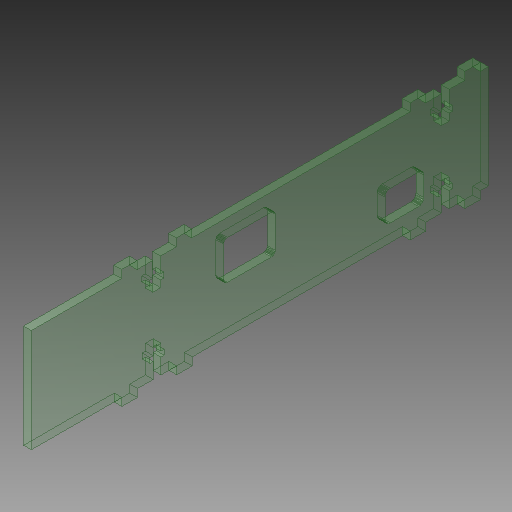
# Autodesk Inventor part: EE Side
Saved by Autodesk Inventor 2018 (Build 220112000, 112)
## iProperties
Created: 2016-07-27
Part Number: EE Side
Material: Polycarbonate, Green
Document SubType Name: Modeling
Designer: User
Density: 1.2 g/cm^3
Appearance: Polycarbonate - Clear(2)
Author: User
Autodesk Inventor part; units mm, degrees
ref_plane "YZ Plane" through (0, 0, 0) normal (1, 0, 0) x (0, 1, 0)
ref_plane "XZ Plane" through (0, 0, 0) normal (0, 1, 0) x (-1, 0, 0)
ref_plane "XY Plane" through (0, 0, 0) normal (0, 0, 1) x (1, 0, 0)
sketch "Sketch1" plane through (0, 0, 0) normal (1, 0, 0) x (0, 1, 0)
  line L0 (104.8297, -51.6375) -> (104.8297, -45.5375)
  line L1 (104.8297, -45.5375) -> (107.8297, -45.5375)
  line L2 (107.8297, -45.5375) -> (107.8297, -39.5375)
  line L3 (107.8297, -39.5375) -> (104.8297, -39.5375)
  line L4 (104.8297, -39.5375) -> (104.8297, -4.6192)
  line L5 (104.8297, -4.6192) -> (64.8298, -4.6192)
  line L6 (64.8298, -4.6192) -> (64.8298, -39.7122)
  line L7 (64.8298, -39.7122) -> (61.8297, -39.7122)
  line L8 (61.8297, -39.7122) -> (61.8297, -45.7122)
  line L9 (61.8297, -45.7122) -> (64.8298, -45.7122)
  line L10 (64.8298, -45.7122) -> (64.8298, -51.8122)
  line L11 (64.8298, -51.8122) -> (70.8298, -51.8122)
  line L12 (70.8298, -51.8122) -> (70.8298, -50.5622)
  line L13 (70.8298, -50.5622) -> (72.8298, -50.5622)
  line L14 (72.8298, -50.5622) -> (72.8298, -51.8122)
  line L15 (72.8298, -51.8122) -> (75.4798, -51.8122)
  line L16 (75.4798, -51.8122) -> (75.4798, -54.8122)
  line L17 (75.4798, -54.8122) -> (72.8298, -54.8122)
  line L18 (72.8298, -54.8122) -> (72.8298, -56.0622)
  line L19 (72.8298, -56.0622) -> (70.8298, -56.0622)
  line L20 (70.8298, -56.0622) -> (70.8298, -54.8122)
  line L21 (70.8298, -54.8122) -> (64.8298, -54.8122)
  line L22 (64.8298, -54.8122) -> (64.8298, -60.9122)
  line L23 (64.8298, -60.9122) -> (61.8297, -60.9122)
  line L24 (61.8297, -60.9122) -> (61.8297, -66.9122)
  line L25 (61.8297, -66.9122) -> (64.8298, -66.9192)
  line L26 (64.8298, -66.9192) -> (64.8298, -67.0192)
  line L27 (64.8298, -67.0192) -> (64.8298, -151.3192)
  line L28 (64.8298, -151.3192) -> (61.8297, -151.3192)
  line L29 (61.8297, -151.3192) -> (61.8297, -157.3192)
  line L30 (61.8297, -157.3192) -> (64.8298, -157.3192)
  line L31 (64.8298, -157.3192) -> (64.8298, -163.4192)
  line L32 (64.8298, -163.4192) -> (70.8298, -163.4192)
  line L33 (70.8298, -163.4192) -> (70.8298, -162.1692)
  line L34 (70.8298, -162.1692) -> (72.8298, -162.1692)
  line L35 (72.8298, -162.1692) -> (72.8298, -163.4192)
  line L36 (72.8298, -163.4192) -> (75.4798, -163.4192)
  line L37 (75.4798, -163.4192) -> (75.4798, -166.4192)
  line L38 (75.4798, -166.4192) -> (72.8298, -166.4192)
  line L39 (72.8298, -166.4192) -> (72.8298, -167.6692)
  line L40 (72.8298, -167.6692) -> (70.8298, -167.6692)
  line L41 (70.8298, -167.6692) -> (70.8298, -166.4192)
  line L42 (70.8298, -166.4192) -> (64.8298, -166.4192)
  line L43 (64.8298, -166.4192) -> (64.8298, -172.5192)
  line L44 (64.8298, -172.5192) -> (61.8297, -172.5192)
  line L45 (61.8297, -172.5192) -> (61.8297, -178.5192)
  line L46 (61.8297, -178.5192) -> (64.8298, -178.5192)
  line L47 (64.8298, -178.5192) -> (64.8298, -178.6192)
  line L48 (64.8298, -178.6192) -> (64.8298, -181.6192)
  line L49 (64.8298, -181.6192) -> (104.8297, -181.6192)
  line L50 (104.8297, -181.6192) -> (104.8297, -178.5192)
  line L51 (104.8297, -178.5192) -> (107.8297, -178.5192)
  line L52 (107.8297, -178.5192) -> (107.8297, -172.5192)
  line L53 (107.8297, -172.5192) -> (104.8297, -172.5192)
  line L54 (104.8297, -172.5192) -> (104.8297, -169.9085)
  line L55 (104.8297, -169.9085) -> (104.8297, -166.4192)
  line L56 (104.8297, -166.4192) -> (98.8297, -166.4192)
  line L57 (98.8297, -166.4192) -> (98.8297, -167.6692)
  line L58 (98.8297, -167.6692) -> (96.8297, -167.6692)
  line L59 (96.8297, -167.6692) -> (96.8297, -166.4192)
  line L60 (96.8297, -166.4192) -> (94.1797, -166.4192)
  line L61 (94.1797, -166.4192) -> (94.1797, -163.4192)
  line L62 (94.1797, -163.4192) -> (96.8297, -163.4192)
  line L63 (96.8297, -163.4192) -> (96.8297, -162.1692)
  line L64 (96.8297, -162.1692) -> (98.8297, -162.1692)
  line L65 (98.8297, -162.1692) -> (98.8297, -163.4192)
  line L66 (98.8297, -163.4192) -> (104.8297, -163.4192)
  line L67 (104.8297, -163.4192) -> (104.8297, -157.3192)
  line L68 (104.8297, -157.3192) -> (107.8297, -157.3192)
  line L69 (107.8297, -157.3192) -> (107.8297, -151.3192)
  line L70 (107.8297, -151.3192) -> (104.8297, -151.3192)
  line L71 (104.8297, -151.3192) -> (104.8297, -66.7375)
  line L72 (104.8297, -66.7375) -> (107.8297, -66.7375)
  line L73 (107.8297, -66.7375) -> (107.8297, -60.7375)
  line L74 (107.8297, -60.7375) -> (104.8297, -60.7375)
  line L75 (104.8297, -60.7375) -> (104.8297, -54.6375)
  line L76 (104.8297, -54.6375) -> (98.8297, -54.6375)
  line L77 (98.8297, -54.6375) -> (98.8297, -55.8875)
  line L78 (98.8297, -55.8875) -> (96.8297, -55.8875)
  line L79 (96.8297, -55.8875) -> (96.8297, -54.6375)
  line L80 (96.8297, -54.6375) -> (94.1797, -54.6375)
  line L81 (94.1797, -54.6375) -> (94.1797, -51.6375)
  line L82 (94.1797, -51.6375) -> (96.8297, -51.6375)
  line L83 (96.8297, -51.6375) -> (96.8297, -50.3875)
  line L84 (96.8297, -50.3875) -> (98.8297, -50.3875)
  line L85 (98.8297, -50.3875) -> (98.8297, -51.6375)
  line L86 (98.8297, -51.6375) -> (104.8297, -51.6375)
  line L87 (82.9657, -143.0778) -> (82.8816, -142.8301)
  line L88 (82.8816, -142.8301) -> (82.7659, -142.5955)
  line L89 (82.7659, -142.5955) -> (82.6206, -142.378)
  line L90 (82.6206, -142.378) -> (82.4481, -142.1813)
  line L91 (82.4481, -142.1813) -> (82.2514, -142.0088)
  line L92 (82.2514, -142.0088) -> (82.0339, -141.8634)
  line L93 (82.0339, -141.8634) -> (81.7993, -141.7477)
  line L94 (81.7993, -141.7477) -> (81.5515, -141.6636)
  line L95 (81.5515, -141.6636) -> (81.0339, -141.5955)
  line L96 (81.0339, -141.5955) -> (73.4376, -141.5955)
  line L97 (73.4376, -141.5955) -> (72.92, -141.6636)
  line L98 (72.92, -141.6636) -> (72.6723, -141.7477)
  line L99 (72.6723, -141.7477) -> (72.4377, -141.8634)
  line L100 (72.4377, -141.8634) -> (72.2202, -142.0088)
  line L101 (72.2202, -142.0088) -> (72.0234, -142.1813)
  line L102 (72.0234, -142.1813) -> (71.851, -142.3779)
  line L103 (71.851, -142.3779) -> (71.7056, -142.5955)
  line L104 (71.7056, -142.5955) -> (71.5899, -142.8301)
  line L105 (71.5899, -142.8301) -> (71.5058, -143.0779)
  line L106 (71.5058, -143.0779) -> (71.4376, -143.5955)
  line L107 (71.4376, -143.5955) -> (71.4376, -154.5955)
  line L108 (71.4376, -154.5955) -> (71.5058, -155.1131)
  line L109 (71.5058, -155.1131) -> (71.5899, -155.3608)
  line L110 (71.5899, -155.3608) -> (71.7056, -155.5955)
  line L111 (71.7056, -155.5955) -> (71.851, -155.813)
  line L112 (71.851, -155.813) -> (72.0234, -156.0097)
  line L113 (72.0234, -156.0097) -> (72.2201, -156.1822)
  line L114 (72.2201, -156.1822) -> (72.4376, -156.3275)
  line L115 (72.4376, -156.3275) -> (72.6723, -156.4432)
  line L116 (72.6723, -156.4432) -> (72.92, -156.5273)
  line L117 (72.92, -156.5273) -> (73.4376, -156.5955)
  line L118 (73.4376, -156.5955) -> (81.0338, -156.5955)
  line L119 (81.0338, -156.5955) -> (81.5515, -156.5273)
  line L120 (81.5515, -156.5273) -> (81.7992, -156.4432)
  line L121 (81.7992, -156.4432) -> (82.0339, -156.3275)
  line L122 (82.0339, -156.3275) -> (82.2514, -156.1822)
  line L123 (82.2514, -156.1822) -> (82.4481, -156.0097)
  line L124 (82.4481, -156.0097) -> (82.6206, -155.813)
  line L125 (82.6206, -155.813) -> (82.7659, -155.5955)
  line L126 (82.7659, -155.5955) -> (82.8816, -155.3608)
  line L127 (82.8816, -155.3608) -> (82.9657, -155.1131)
  line L128 (82.9657, -155.1131) -> (83.0339, -154.5955)
  line L129 (83.0339, -154.5955) -> (83.0339, -149.0956)
  line L130 (83.0339, -149.0956) -> (83.0339, -143.5955)
  line L131 (83.0339, -143.5955) -> (82.9657, -143.0778)
  line L132 (97.9828, -80.2073) -> (97.9197, -80.0215)
  line L133 (97.9197, -80.0215) -> (97.8329, -79.8455)
  line L134 (97.8329, -79.8455) -> (97.7239, -79.6823)
  line L135 (97.7239, -79.6823) -> (97.5945, -79.5348)
  line L136 (97.5945, -79.5348) -> (97.447, -79.4055)
  line L137 (97.447, -79.4055) -> (97.2839, -79.2964)
  line L138 (97.2839, -79.2964) -> (97.1079, -79.2097)
  line L139 (97.1079, -79.2097) -> (96.9221, -79.1466)
  line L140 (96.9221, -79.1466) -> (96.5339, -79.0955)
  line L141 (96.5339, -79.0955) -> (84.5339, -79.0955)
  line L142 (84.5339, -79.0955) -> (84.1457, -79.1466)
  line L143 (84.1457, -79.1466) -> (83.9599, -79.2097)
  line L144 (83.9599, -79.2097) -> (83.7839, -79.2964)
  line L145 (83.7839, -79.2964) -> (83.6207, -79.4055)
  line L146 (83.6207, -79.4055) -> (83.4732, -79.5348)
  line L147 (83.4732, -79.5348) -> (83.3439, -79.6823)
  line L148 (83.3439, -79.6823) -> (83.2348, -79.8454)
  line L149 (83.2348, -79.8454) -> (83.1481, -80.0215)
  line L150 (83.1481, -80.0215) -> (83.085, -80.2072)
  line L151 (83.085, -80.2072) -> (83.0339, -80.5955)
  line L152 (83.0339, -80.5955) -> (83.0339, -89.0955)
  line L153 (83.0339, -89.0955) -> (83.0339, -97.5955)
  line L154 (83.0339, -97.5955) -> (83.085, -97.9837)
  line L155 (83.085, -97.9837) -> (83.1481, -98.1695)
  line L156 (83.1481, -98.1695) -> (83.2348, -98.3455)
  line L157 (83.2348, -98.3455) -> (83.3439, -98.5086)
  line L158 (83.3439, -98.5086) -> (83.4732, -98.6562)
  line L159 (83.4732, -98.6562) -> (83.6207, -98.7855)
  line L160 (83.6207, -98.7855) -> (83.7839, -98.8945)
  line L161 (83.7839, -98.8945) -> (83.9598, -98.9813)
  line L162 (83.9598, -98.9813) -> (84.1456, -99.0444)
  line L163 (84.1456, -99.0444) -> (84.5339, -99.0955)
  line L164 (84.5339, -99.0955) -> (96.5339, -99.0955)
  line L165 (96.5339, -99.0955) -> (96.9221, -99.0444)
  line L166 (96.9221, -99.0444) -> (97.1079, -98.9813)
  line L167 (97.1079, -98.9813) -> (97.2839, -98.8945)
  line L168 (97.2839, -98.8945) -> (97.447, -98.7855)
  line L169 (97.447, -98.7855) -> (97.5946, -98.6562)
  line L170 (97.5946, -98.6562) -> (97.7239, -98.5087)
  line L171 (97.7239, -98.5087) -> (97.8329, -98.3456)
  line L172 (97.8329, -98.3456) -> (97.9197, -98.1696)
  line L173 (97.9197, -98.1696) -> (97.9828, -97.9838)
  line L174 (97.9828, -97.9838) -> (98.0339, -97.5957)
  line L175 (98.0339, -97.5957) -> (98.0339, -80.5957)
  line L176 (98.0339, -80.5957) -> (97.9828, -80.2073)
  point P0 (0, 0)
  constraints: 354 end point, 94 parallel, 68 perpendicular, 2 collinear
extrude "Extrusion1" add sketch "Sketch1" along normal blind 3
body "Solid1"
